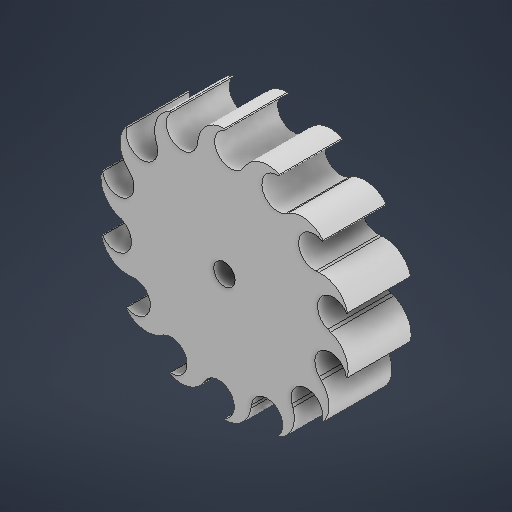
# Autodesk Inventor part: Turbine
Saved by Autodesk Inventor 2025.3 (Build 293356030, 356C)
## iProperties
Created: 2025-09-28
Part Number: Turbine
Material: Generic
Document SubType Name: Modeling
Designer: yo
Density: 1 g/cm^3
Appearance: Default
Author: yo
Autodesk Inventor part; units mm, degrees
ref_plane "YZ Plane" through (0, 0, 0) normal (1, 0, 0) x (0, 1, 0)
ref_plane "XZ Plane" through (0, 0, 0) normal (0, 1, 0) x (-1, 0, 0)
ref_plane "XY Plane" through (0, 0, 0) normal (0, 0, 1) x (1, 0, 0)
sketch "Sketch1" plane through (0, 0, 0) normal (0, 0, 1) x (1, 0, 0)
  circle A0 centre (0, 0) radius 40 construction
  circle A1 centre (0, 0) radius 30 construction
  arc A2 (0.0721, 39.6135) -> (0, 40) centre (0, 39.8) ccw
  arc A3 (0.0721, 39.6135) -> (6.0648, 32.2214) centre (1.8749, 34.9497) ccw
  line L0 (6.0648, 32.2214) -> (6.5929, 33.0323)
  line L1 (1.607, 29.9569) -> (7.607, 29.6351) construction
  arc A4 (0, 40) -> (-8.3922, 32.6216) centre (0, 31.5381) ccw
  arc A5 (-17.1227, 35.7218) -> (-17.3553, 36.0388) centre (-17.2686, 35.8586) ccw
  arc A6 (-17.1227, 35.7218) -> (-8.5161, 31.6619) centre (-13.4749, 32.3021) ccw
  line L2 (-8.5161, 31.6619) -> (-8.3922, 32.6216)
  arc A7 (-17.3553, 36.0388) -> (-21.7151, 25.7498) centre (-13.6839, 28.4149) ccw
  arc A8 (-30.9261, 24.755) -> (-31.2733, 24.9396) centre (-31.1169, 24.8149) ccw
  arc A9 (-30.9261, 24.755) -> (-21.4103, 24.8314) centre (-26.1559, 23.2566) ccw
  line L3 (-21.4103, 24.8314) -> (-21.7151, 25.7498)
  arc A10 (-31.2733, 24.9396) -> (-30.7371, 13.778) centre (-24.6575, 19.6637) ccw
  arc A11 (-38.6042, 8.8851) -> (-38.9971, 8.9008) centre (-38.8021, 8.8563) ccw
  arc A12 (-38.6042, 8.8851) -> (-30.064, 13.0827) centre (-33.6563, 9.6049) ccw
  line L4 (-30.064, 13.0827) -> (-30.7371, 13.778)
  arc A13 (-38.9971, 8.9008) -> (-33.6712, -0.9228) centre (-30.7474, 7.0179) ccw
  arc A14 (-38.6363, -8.7445) -> (-38.9971, -8.9008) centre (-38.8021, -8.8563) ccw
  arc A15 (-38.6363, -8.7445) -> (-32.7631, -1.2571) centre (-34.4907, -5.9492) ccw
  line L5 (-32.7631, -1.2571) -> (-33.6712, -0.9228)
  arc A16 (-38.9971, -8.9008) -> (-29.9363, -15.4408) centre (-30.7474, -7.0179) ccw
  arc A17 (-31.016, -24.6422) -> (-31.2733, -24.9396) centre (-31.1169, -24.8149) ccw
  arc A18 (-31.016, -24.6422) -> (-28.9731, -15.348) centre (-28.4938, -20.325) ccw
  line L6 (-28.9731, -15.348) -> (-29.9363, -15.4408)
  arc A19 (-31.2733, -24.9396) -> (-20.2721, -26.9005) centre (-24.6575, -19.6637) ccw
  arc A20 (-17.2526, -35.6592) -> (-17.3553, -36.0388) centre (-17.2686, -35.8586) ccw
  arc A21 (-17.2526, -35.6592) -> (-19.4446, -26.399) centre (-16.8533, -30.6752) ccw
  line L7 (-19.4446, -26.399) -> (-20.2721, -26.9005)
  arc A22 (-17.3553, -36.0388) -> (-6.5929, -33.0323) centre (-13.6839, -28.4149) ccw
  arc A23 (-0.0721, -39.6135) -> (0, -40) centre (0, -39.8) ccw
  arc A24 (-0.0721, -39.6135) -> (-6.0648, -32.2214) centre (-1.8749, -34.9497) ccw
  line L8 (-6.0648, -32.2214) -> (-6.5929, -33.0323)
  arc A25 (0, -40) -> (8.3922, -32.6216) centre (0, -31.5381) ccw
  arc A26 (17.1227, -35.7218) -> (17.3553, -36.0388) centre (17.2686, -35.8586) ccw
  arc A27 (17.1227, -35.7218) -> (8.5161, -31.6619) centre (13.4749, -32.3021) ccw
  line L9 (8.5161, -31.6619) -> (8.3922, -32.6216)
  arc A28 (17.3553, -36.0388) -> (21.7151, -25.7498) centre (13.6839, -28.4149) ccw
  arc A29 (30.9261, -24.755) -> (31.2733, -24.9396) centre (31.1169, -24.8149) ccw
  arc A30 (30.9261, -24.755) -> (21.4103, -24.8314) centre (26.1559, -23.2566) ccw
  line L10 (21.4103, -24.8314) -> (21.7151, -25.7498)
  arc A31 (31.2733, -24.9396) -> (30.7371, -13.778) centre (24.6575, -19.6637) ccw
  arc A32 (38.6042, -8.8851) -> (38.9971, -8.9008) centre (38.8021, -8.8563) ccw
  arc A33 (38.6042, -8.8851) -> (30.064, -13.0827) centre (33.6563, -9.6049) ccw
  line L11 (30.064, -13.0827) -> (30.7371, -13.778)
  arc A34 (38.9971, -8.9008) -> (33.6712, 0.9228) centre (30.7474, -7.0179) ccw
  arc A35 (38.6363, 8.7445) -> (38.9971, 8.9008) centre (38.8021, 8.8563) ccw
  arc A36 (38.6363, 8.7445) -> (32.7631, 1.2571) centre (34.4907, 5.9492) ccw
  line L12 (32.7631, 1.2571) -> (33.6712, 0.9228)
  arc A37 (38.9971, 8.9008) -> (29.9363, 15.4408) centre (30.7474, 7.0179) ccw
  arc A38 (31.016, 24.6422) -> (31.2733, 24.9396) centre (31.1169, 24.8149) ccw
  arc A39 (31.016, 24.6422) -> (28.9731, 15.348) centre (28.4938, 20.325) ccw
  line L13 (28.9731, 15.348) -> (29.9363, 15.4408)
  arc A40 (31.2733, 24.9396) -> (20.2721, 26.9005) centre (24.6575, 19.6637) ccw
  arc A41 (17.2526, 35.6592) -> (17.3553, 36.0388) centre (17.2686, 35.8586) ccw
  arc A42 (17.2526, 35.6592) -> (19.4446, 26.399) centre (16.8533, 30.6752) ccw
  line L14 (19.4446, 26.399) -> (20.2721, 26.9005)
  arc A43 (17.3553, 36.0388) -> (6.5929, 33.0323) centre (13.6839, 28.4149) ccw
  circle A44 centre (0, 0) radius 3.4
  point P0 (-11.55, 27.6875)
  point P1 (-22.4193, 19.9343)
  point P2 (-28.8483, 8.2328)
  point P3 (-29.5634, -5.0993)
  point P4 (-24.4232, -17.4214)
  point P5 (-14.4457, -26.293)
  point P6 (-1.607, -29.9569)
  point P7 (11.55, -27.6875)
  point P8 (22.4193, -19.9343)
  point P9 (28.8483, -8.2328)
  point P10 (29.5634, 5.0993)
  point P11 (24.4232, 17.4214)
  point P12 (14.4457, 26.293)
  point P13 (-8.3922, 32.6216)
  point P14 (-21.7151, 25.7498)
  point P15 (-30.7371, 13.778)
  point P16 (-33.6712, -0.9228)
  point P17 (-29.9363, -15.4408)
  point P18 (-6.5929, -33.0323)
  point P19 (8.3922, -32.6216)
  point P20 (30.7371, -13.778)
  point P21 (33.6712, 0.9228)
  point P22 (29.9363, 15.4408)
  point P23 (20.2721, 26.9005)
  dimension "d14" = 60
  dimension "d6" = 80
  dimension "d16" = 0.2
  dimension "d22" = 5
  dimension "d23" = 60
  dimension "d28" = 6
  dimension "d31" = 360
  dimension "d33" = 6.8
  constraints: 98 point on circle, 44 centre point, 30 end point, 7 tangent, 4 coincident, 2 vertical alignment, 188 other
  measures "d6" diameter of A0
  measures "d16" radius of A2
  measures "d22" radius of A3
  measures "d23" angle of L1 L0
  measures "d28" horizontal distance of L1.start L1.end
  measures "d33" diameter of A44
extrude "Extrusion1" add sketch "Sketch1" along normal mid plane 20
body "Solid1"
